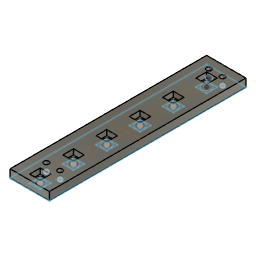
4Sight EV7 Bracket v7 (Autodesk Fusion 360 design; units mm, degrees)
Autodesk Fusion 360 part; units mm, degrees
sketch "Schizzo1" plane through (0, 0, 0) normal (0, 0, 1) x (1, 0, 0)
  line L0 (25.7791, 75.2827) -> (55.7791, 75.2827)
  line L1 (55.7791, 75.2827) -> (55.7791, -74.7173)
  line L2 (55.7791, -74.7173) -> (25.7791, -74.7173)
  line L3 (25.7791, -74.7173) -> (25.7791, 75.2827)
  line L4 (40.7791, 75.2827) -> (40.7791, -74.7173) construction
  line L5 (25.7791, 0.2827) -> (55.7791, 0.2827) construction
  circle A0 centre (40.7791, 60.2827) radius 3.4
  line L6 (44.8291, 56.2327) -> (36.7291, 56.2327)
  line L7 (36.7291, 56.2327) -> (36.7291, 64.3327)
  line L8 (36.7291, 64.3327) -> (44.8291, 64.3327)
  line L9 (44.8291, 64.3327) -> (44.8291, 56.2327)
  line L10 (44.8291, 56.2327) -> (36.7291, 64.3327) construction
  line L11 (36.7291, 56.2327) -> (44.8291, 64.3327) construction
  line L12 (44.8291, 38.9327) -> (44.8291, 30.8327)
  line L13 (36.7291, 38.9327) -> (44.8291, 38.9327)
  line L14 (36.7291, 30.8327) -> (36.7291, 38.9327)
  circle A1 centre (40.7791, 34.8827) radius 3.4
  line L15 (44.8291, 30.8327) -> (36.7291, 30.8327)
  line L16 (44.8291, 13.5327) -> (44.8291, 5.4327)
  line L17 (36.7291, 13.5327) -> (44.8291, 13.5327)
  line L18 (36.7291, 5.4327) -> (36.7291, 13.5327)
  circle A2 centre (40.7791, 9.4827) radius 3.4
  line L19 (44.8291, 5.4327) -> (36.7291, 5.4327)
  line L20 (44.8291, -11.8673) -> (44.8291, -19.9673)
  line L21 (36.7291, -11.8673) -> (44.8291, -11.8673)
  line L22 (36.7291, -19.9673) -> (36.7291, -11.8673)
  circle A3 centre (40.7791, -15.9173) radius 3.4
  line L23 (44.8291, -19.9673) -> (36.7291, -19.9673)
  line L24 (44.8291, -37.2673) -> (44.8291, -45.3673)
  line L25 (36.7291, -37.2673) -> (44.8291, -37.2673)
  line L26 (36.7291, -45.3673) -> (36.7291, -37.2673)
  circle A4 centre (40.7791, -41.3173) radius 3.4
  line L27 (44.8291, -45.3673) -> (36.7291, -45.3673)
  line L28 (44.8291, -62.6673) -> (44.8291, -70.7673)
  line L29 (36.7291, -62.6673) -> (44.8291, -62.6673)
  line L30 (36.7291, -70.7673) -> (36.7291, -62.6673)
  circle A5 centre (40.7791, -66.7173) radius 3.4
  line L31 (44.8291, -70.7673) -> (36.7291, -70.7673)
  line L32 (35.5791, 75.2827) -> (35.5791, -74.7173) construction
  circle A6 centre (35.5791, 67.2827) radius 1.9
  circle A7 centre (45.9791, 67.2827) radius 1.9
  circle A8 centre (35.5791, -56.7173) radius 1.9
  circle A9 centre (45.9791, -56.7173) radius 1.9
  point P0 (40.7791, 60.2827)
  dimension "d1" = 30
  dimension "d2" = 150
  dimension "d3" = 6.8
  dimension "d4" = 8.1
  dimension "d5" = 8.1
  dimension "d8" = 25.4
  dimension "d9" = 0
  dimension "d11" = 15
  dimension "d22" = 5.2
  dimension "d23" = 3.8
  dimension "d24" = 8
  dimension "d27" = 124
  dimension "d28" = 0
  dimension "d29" = 25.4
  dimension "d30" = 124
  constraint horizontal L0
  constraint vertical L1
  constraint horizontal L2
  constraint vertical L3
  constraint midpoint L0 L4.start
  constraint midpoint L2 L4.end
  constraint midpoint L3 L5.start
  constraint midpoint L1 L5.end
  constraint coincident L4 P0
  constraint horizontal L6
  constraint perpendicular L6 L7
  constraint parallel L6 L8
  constraint parallel L7 L9
  constraint coincident L10 P0
  constraint coincident L11 P0
  constraint coincident P0 A0.centre
  constraint coincident L0 L32.start
  constraint coincident L2 L32.end
  constraint perpendicular L2 L32
  constraint coincident L32 A6.centre
  constraint symmetric L4 A6 A7
  measures "d1" distance of L0.start L0.end
  measures "d2" distance of L0.start L2.end
  measures "d3" diameter of A0
  measures "d4" distance of L7.end L8.end
  measures "d5" distance of L6.end L7.end
  measures "d11" distance of L0 P0
  measures "d22" distance of L4 L32
  measures "d23" diameter of A6
  measures "d24" distance of L0 A6.centre
  measures "d29" distance of L15 L19
  measures "d30" distance of A6.centre A8.centre
extrude "Estrusione1" add sketch "Schizzo1" along normal blind 6 contours L0 L1 L2 L3
extrude "Estrusione2" add sketch "Schizzo1" along normal blind 2 contours L6 L7 L8 L9 | L12 L13 L14 L15 | L16 L17 L18 L19 | L20 L21 L22 L23 | L24 L25 L26 L27 | L28 L29 L30 L31
